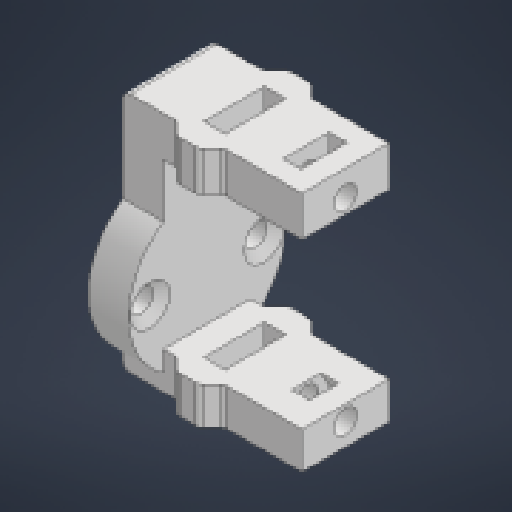
# Autodesk Inventor part: sg90 claw v2 holder
Saved by Autodesk Inventor 2026.1 (Build 301233020, 233B)
## iProperties
Created: 2025-05-12
Part Number: sg90 claw v2 holder
Material: 一般
Document SubType Name: Modeling
Designer: gavin
Density: 1 g/cm^3
Appearance: 預設
Author: gavin
## iProperties of the stored document sg90 claw v2 holder_3D 列印.ipt
Created: 2025-05-12
Part Number: sg90 claw v2 holder_3D 列印
Material: 一般
Document SubType Name: Modeling
Designer: gavin
Density: 1 g/cm^3
Appearance: 預設
Author: gavin
Autodesk Inventor part; units mm, degrees
ref_plane "YZ Plane" through (0, 0, 0) normal (1, 0, 0) x (0, 1, 0)
ref_plane "XZ Plane" through (0, 0, 0) normal (0, 1, 0) x (-1, 0, 0)
ref_plane "XY Plane" through (0, 0, 0) normal (0, 0, 1) x (1, 0, 0)
sketch "草圖1" plane through (0, 0, 0) normal (0, 0, 1) x (1, 0, 0)
  line L0 (-4.2926, 4.2164) -> (-4.2926, -0.635) projected
  line L1 (-4.2926, 4.2164) -> (-6.6548, 4.2164) projected
  line L2 (-6.6548, 4.2164) -> (-6.6548, -0.635) projected
  line L3 (-6.6548, -0.635) -> (-22.225, -0.635) projected
  line L4 (-22.225, -0.635) -> (-22.225, -3.6963) construction
  line L5 (-22.225, -3.6963) -> (-23.241, -3.6963) construction
  line L6 (-23.241, -3.6963) -> (-23.241, -19.2054) construction
  line L7 (-23.241, -19.2054) -> (-21.209, -19.2054) construction
  line L8 (-21.209, -19.2054) -> (-21.209, -21.9456) construction
  line L9 (-21.209, -21.9456) -> (-6.6548, -21.9456) projected
  line L10 (-6.6548, -26.797) -> (-6.6548, -21.9456) construction
  line L11 (-6.6548, -26.797) -> (-4.2926, -26.797) construction
  line L12 (-4.2926, -26.797) -> (-4.2926, -21.9456) projected
  line L13 (-4.2926, -21.9456) -> (0, -21.9456) projected
  line L14 (0, -16.4846) -> (0, -21.9456) projected
  line L15 (0, -0.635) -> (0, -16.4846) projected
  line L16 (0, -0.635) -> (-4.2926, -0.635) projected
  line L17 (-6.6548, -19.8311) -> (-6.6548, -2.7496) projected
  line L18 (-19.6088, -19.8311) -> (-6.6548, -19.8311) projected
  line L19 (-19.6088, -2.7496) -> (-19.6088, -19.8311) projected
  line L20 (-6.6548, -2.7496) -> (-19.6088, -2.7496) projected
  line L21 (-23.06, 0.2) -> (-12.0824, 0.2)
  line L22 (-6.8548, 4.8514) -> (-6.6548, 4.8514)
  line L23 (-4.0926, 4.4164) -> (-4.0926, -0.435)
  line L24 (-4.0926, -0.435) -> (0.2, -0.435)
  line L25 (0.2, -0.435) -> (0.2, -16.4846)
  line L26 (0.2, -16.4846) -> (0.2, -22.1456)
  line L27 (0.2, -22.1456) -> (-4.0926, -22.1456)
  line L28 (-4.0926, -22.1456) -> (-4.0926, -26.997)
  line L29 (-6.6548, -26.997) -> (-9.1539, -26.997)
  line L30 (-6.8548, -22.7806) -> (-22.044, -22.7806)
  line L31 (-22.044, -22.7806) -> (-22.044, -20.0404) construction
  line L32 (-22.044, -20.0404) -> (-24.076, -20.0404) construction
  line L33 (-24.076, -20.0404) -> (-24.076, -2.8613) construction
  line L34 (-24.076, -2.8613) -> (-23.06, -2.8613) construction
  line L35 (-23.06, -2.8613) -> (-23.06, 0.2) construction
  line L36 (-6.8548, 4.8514) -> (-31.7274, 4.8514)
  line L37 (-24.076, -11.4509) -> (-24.6908, -11.4509)
  line L38 (-31.7274, 4.8514) -> (-31.7274, -11.4509)
  line L39 (-23.06, 0.2) -> (-27.076, 0.2)
  line L40 (-27.076, 0.2) -> (-27.076, -11.4509)
  line L41 (-9.1539, -26.997) -> (-31.7274, -26.997)
  line L42 (-31.7274, -26.997) -> (-31.7274, -11.4509)
  line L43 (-27.076, -11.4509) -> (-27.076, -22.7806)
  line L44 (-27.076, -22.7806) -> (-22.044, -22.7806)
  line L45 (-6.6548, 4.8514) -> (-6.6548, 0.2)
  line L46 (-12.0824, 0.2) -> (-6.6548, 0.2)
  line L47 (-6.8548, -22.7806) -> (-6.6548, -22.7806)
  line L48 (-6.6548, -26.997) -> (-6.6548, -22.7806)
  line L49 (-6.6548, -22.5806) -> (-21.844, -22.5806)
  line L50 (-22.225, 0) -> (-6.6548, 0)
  line L51 (-6.6548, 4.8514) -> (-4.2926, 4.8514)
  point P0 (0, 0)
  point P1 (-5.4737, 4.8514)
  dimension "d4" = 3
  dimension "d6" = 4.6514
  dimension "d7" = 4.6514
  dimension "d37" = 0.2
  dimension "d38" = 0.2
  constraints: 62 end point, 7 horizontal, 5 perpendicular, 5 point on line, 3 vertical, 2 collinear, 2 midpoint, 1 horizontal alignment, 16 other
  measures "d4" distance between parallel lines of L40 L33
  measures "d6" distance between parallel lines of L39 L36
  measures "d7" distance between parallel lines of L38 L40
  measures "d37" distance between parallel lines of L50 L21
  measures "d38" distance between parallel lines of L49 L30
ref_plane "工作平面1" through (-23.241, -26.797, -12.192) normal (0, 0, -1) x (0, 1, 0)
extrude "擠出1" add sketch "草圖1" against normal up to surface (12.192 mm away) contours L2 L46 L21 L39 L40 L43 L44 L30 L47 L48 L29 L41 L42 L38 L36 L22 L45
sketch "草圖3" plane through (-31.7274, 4.8514, 0) normal (0, 1, 0) x (1, 0, 0)
  line L0 (25.0726, 12.192) -> (0, 12.192) projected
  line L1 (0, 0) -> (0, 12.192) projected
  line L2 (25.0726, 0) -> (0, 0) projected
  line L3 (25.0726, 0) -> (25.0726, 12.192) projected
  point P0 (31.7274, 0)
extrude "擠出3" add sketch "草圖3" along normal blind 1
sketch "草圖4" plane through (-31.7274, -26.997, 0) normal (0, -1, 0) x (1, 0, 0)
  line L0 (0, -12.192) -> (25.0726, -12.192) projected
  line L1 (0, 0) -> (25.0726, 0) projected
  line L2 (0, 0) -> (0, -12.192) projected
  line L3 (25.0726, 0) -> (25.0726, -12.192) projected
  point P0 (31.7274, 0)
extrude "擠出4" add sketch "草圖4" along normal blind 1
ref_plane "工作平面2" through (-9.6548, -22.7806, 0) normal (1, 0, 0) x (0, 0, -1)
sketch "草圖5" plane through (-9.6548, -22.7806, 0) normal (1, 0, 0) x (0, 0, -1)
  circle A0 centre (6.096, -2.086) radius 1.65 projected
  line L0 (4.4794, -4.886) -> (2.8628, -2.086)
  line L1 (2.8628, -2.086) -> (4.4794, 0.714)
  line L2 (4.4794, 0.714) -> (7.7126, 0.714)
  line L3 (7.7126, 0.714) -> (9.3292, -2.086)
  line L4 (9.3292, -2.086) -> (7.7126, -4.886)
  line L5 (7.7126, -4.886) -> (4.4794, -4.886)
  line L6 (2.8628, -2.086) -> (2.8628, -8.9822)
  line L7 (2.8628, -8.9822) -> (9.3292, -8.9822)
  line L8 (9.3292, -8.9822) -> (9.3292, -2.086)
  point P0 (0, 22.7806)
  dimension "d19" = 5.6
  constraints: 18 end point, 2 perpendicular, 1 coincident, 1 vertical, 13 other
  measures "d19" distance between parallel lines of L5 L2
extrude "擠出5" cut sketch "草圖5" against normal blind 2.5 contours A0 | L5 L4 L8 L7 L6 L0 | L0 L1 L2 L3 L4 L5
ref_plane "工作平面3" through (-31.7274, -11.0728, 0) normal (0, 1, 0) x (1, 0, 0)
mirror "鏡射1" about plane through (-31.7274, -11.0728, 0) normal (0, 1, 0) of "擠出5"
sketch "草圖10" plane through (-6.6548, -22.7806, 0) normal (1, 0, 0) x (0, 0, -1)
  circle A0 centre (6.096, 25.0666) radius 1.6 projected
  arc A1 (6.731, -3.8821) -> (5.461, -3.8821) centre (6.096, -2.086) ccw projected
  circle A2 centre (6.096, -2.086) radius 1.65
  circle A3 centre (6.096, 25.0666) radius 1.65
  point P0 (0, 22.7806)
  dimension "d39" = 3.3
  dimension "d40" = 3.3
  constraints: 2 centre point, 1 coincident
  measures "d39" diameter of A2
  measures "d40" diameter of A3
extrude "擠出10" cut sketch "草圖10" against normal blind 11 contours A0 | A2
fillet "圓角2" radius 1 1 edges at (-31.7274, 5.8514, -6.096)
sketch "草圖12" plane through (-31.7274, 5.8514, 0) normal (0, 1, 0) x (1, 0, 0)
  line L0 (1, 0) -> (1, 12.192) projected
  line L1 (1, 0) -> (25.0726, 0) projected
  line L2 (25.0726, 0) -> (25.0726, 12.192) projected
  line L3 (25.0726, 12.192) -> (1, 12.192) projected
  line L4 (19.5726, 9.3292) -> (22.0726, 9.3292) projected
  line L5 (22.0726, 9.3292) -> (22.0726, 2.8628) projected
  line L6 (22.0726, 2.8628) -> (19.5726, 2.8628) projected
  line L7 (19.5726, 2.8628) -> (19.5726, 9.3292) projected
  line L8 (12.4726, 10.346) -> (9.4726, 10.346)
  line L9 (9.4726, 10.346) -> (9.4726, 1.846)
  line L10 (9.4726, 1.846) -> (12.4726, 1.846)
  line L11 (12.4726, 1.846) -> (12.4726, 10.346)
  point P0 (31.7274, 0)
  dimension "d47" = 3
  dimension "d48" = 8.5
  dimension "d49" = 12.192
  dimension "d50" = 1.846
  dimension "d51" = 12.6
  constraints: 8 end point, 2 parallel, 1 horizontal, 1 perpendicular
  measures "d47" distance of L9.end L10.end
  measures "d48" distance of L8.end L9.end
  measures "d49" distance of L1.end L2.end
  measures "d50" distance between parallel lines of L8 L3
  measures "d51" distance between parallel lines of L2 L11
extrude "擠出12" cut sketch "草圖12" against normal up to surface (5.6514 mm away) contours L11 L10 L9 L8
sketch "草圖13" plane through (-31.7274, 5.8514, 0) normal (0, 1, 0) x (1, 0, 0)
  line L0 (9.4726, 10.346) -> (12.4726, 10.346) projected
  line L1 (12.4726, 10.346) -> (12.4726, 1.846) projected
  line L2 (12.4726, 1.846) -> (9.4726, 1.846) projected
  line L3 (9.4726, 1.846) -> (9.4726, 10.346) projected
  line L4 (1, 0) -> (1, 12.192) projected
  line L5 (1, 0) -> (25.0726, 0) projected
  line L6 (25.0726, 0) -> (25.0726, 12.192) projected
  line L7 (25.0726, 12.192) -> (1, 12.192) projected
  line L8 (19.5726, 9.3292) -> (22.0726, 9.3292) projected
  line L9 (22.0726, 9.3292) -> (22.0726, 2.8628) projected
  line L10 (22.0726, 2.8628) -> (19.5726, 2.8628) projected
  line L11 (19.5726, 2.8628) -> (19.5726, 9.3292) projected
  line L12 (12.3526, 13.992) -> (9.3526, 13.992)
  line L13 (9.3526, 13.992) -> (7.5526, 12.192)
  line L14 (12.3526, 13.992) -> (14.1526, 12.192)
  line L15 (25.0726, 6.096) -> (20.8226, 6.096) construction
  line L16 (12.3526, -1.8) -> (9.3526, -1.8)
  line L17 (9.3526, -1.8) -> (7.5526, 0)
  line L18 (12.3526, -1.8) -> (14.1526, 0)
  point P0 (31.7274, 0)
  dimension "d54" = 135
  dimension "d55" = 135
  dimension "d56" = 1.8
  constraints: 14 end point, 4 symmetric about line, 2 horizontal, 2 point on line, 1 midpoint
  measures "d54" angle of L12 L14
  measures "d55" angle of L13 L12
  measures "d56" distance between parallel lines of L7 L12
extrude "擠出13" add sketch "草圖13" against normal up to surface (5.6514 mm away) contours L5 L18 L16 L17 | L13 L12 L14 L7
fillet "圓角3" radius 1 8 edges at (-17.5748, 3.0257, 0) (-19.3748, 3.0257, 1.8) (-22.3748, 3.0257, 1.8) (-24.1748, 3.0257, 0) (-17.5748, 3.0257, -12.192) (-19.3748, 3.0257, -13.992) (-22.3748, 3.0257, -13.992) (-24.1748, 3.0257, -12.192)
sketch "草圖14" plane through (-31.7274, -27.997, 0) normal (0, -1, 0) x (1, 0, 0)
  line L0 (12.4726, -10.346) -> (9.4726, -10.346) projected
  line L1 (9.4726, -10.346) -> (9.4726, -1.846) projected
  line L2 (9.4726, -1.846) -> (12.4726, -1.846) projected
  line L3 (12.4726, -1.846) -> (12.4726, -10.346) projected
  line L4 (22.0726, -7.8737) -> (19.5726, -7.8737) projected
  line L5 (19.5726, -7.8737) -> (19.5726, -4.3183) projected
  line L6 (19.5726, -4.3183) -> (22.0726, -4.3183) projected
  line L7 (22.0726, -4.3183) -> (22.0726, -7.8737) projected
  arc A0 (9.0597, -13.6991) -> (9.7668, -13.992) centre (9.7668, -12.992) ccw projected
  line L8 (11.9384, -13.992) -> (9.7668, -13.992) projected
  arc A1 (11.9384, -13.992) -> (12.6455, -13.6991) centre (11.9384, -12.992) ccw projected
  line L9 (13.8597, -12.4849) -> (12.6455, -13.6991) projected
  arc A2 (14.5668, -12.192) -> (13.8597, -12.4849) centre (14.5668, -13.192) ccw projected
  line L10 (14.5668, -12.192) -> (25.0726, -12.192) projected
  line L11 (25.0726, 0) -> (25.0726, -12.192) projected
  line L12 (14.5668, 0) -> (25.0726, 0) projected
  arc A3 (13.8597, 0.2929) -> (14.5668, 0) centre (14.5668, 1) ccw projected
  line L13 (12.6455, 1.5071) -> (13.8597, 0.2929) projected
  arc A4 (12.6455, 1.5071) -> (11.9384, 1.8) centre (11.9384, 0.8) ccw projected
  line L14 (9.7668, 1.8) -> (11.9384, 1.8) projected
  arc A5 (9.7668, 1.8) -> (9.0597, 1.5071) centre (9.7668, 0.8) ccw projected
  line L15 (7.8455, 0.2929) -> (9.0597, 1.5071) projected
  arc A6 (7.1384, 0) -> (7.8455, 0.2929) centre (7.1384, 1) ccw projected
  line L16 (4.6514, 0) -> (7.1384, 0) projected
  line L17 (4.6514, 0) -> (4.6514, -12.192) projected
  line L18 (4.6514, -12.192) -> (7.1384, -12.192) projected
  arc A7 (7.8455, -12.4849) -> (7.1384, -12.192) centre (7.1384, -13.192) ccw projected
  line L19 (9.0597, -13.6991) -> (7.8455, -12.4849) projected
  point P0 (31.7274, 0)
extrude "擠出14" cut sketch "草圖14" against normal up to surface (5.2164 mm away) contours L0 L1 L2 L3
sketch "草圖15" plane through (-31.7274, -27.997, 0) normal (0, -1, 0) x (1, 0, 0)
  line L0 (12.4726, -10.346) -> (9.4726, -10.346) projected
  line L1 (9.4726, -10.346) -> (9.4726, -1.846) projected
  line L2 (9.4726, -1.846) -> (12.4726, -1.846) projected
  line L3 (12.4726, -1.846) -> (12.4726, -10.346) projected
  line L4 (22.0726, -7.8737) -> (19.5726, -7.8737) projected
  line L5 (19.5726, -7.8737) -> (19.5726, -4.3183) projected
  line L6 (19.5726, -4.3183) -> (22.0726, -4.3183) projected
  line L7 (22.0726, -4.3183) -> (22.0726, -7.8737) projected
  arc A0 (9.0597, -13.6991) -> (9.7668, -13.992) centre (9.7668, -12.992) ccw projected
  line L8 (11.9384, -13.992) -> (9.7668, -13.992) projected
  arc A1 (11.9384, -13.992) -> (12.6455, -13.6991) centre (11.9384, -12.992) ccw projected
  line L9 (13.8597, -12.4849) -> (12.6455, -13.6991) projected
  arc A2 (14.5668, -12.192) -> (13.8597, -12.4849) centre (14.5668, -13.192) ccw projected
  line L10 (14.5668, -12.192) -> (25.0726, -12.192) projected
  line L11 (25.0726, 0) -> (25.0726, -12.192) projected
  line L12 (14.5668, 0) -> (25.0726, 0) projected
  arc A3 (13.8597, 0.2929) -> (14.5668, 0) centre (14.5668, 1) ccw projected
  line L13 (12.6455, 1.5071) -> (13.8597, 0.2929) projected
  arc A4 (12.6455, 1.5071) -> (11.9384, 1.8) centre (11.9384, 0.8) ccw projected
  line L14 (9.7668, 1.8) -> (11.9384, 1.8) projected
  arc A5 (9.7668, 1.8) -> (9.0597, 1.5071) centre (9.7668, 0.8) ccw projected
  line L15 (7.8455, 0.2929) -> (9.0597, 1.5071) projected
  arc A6 (7.1384, 0) -> (7.8455, 0.2929) centre (7.1384, 1) ccw projected
  line L16 (4.6514, 0) -> (7.1384, 0) projected
  line L17 (4.6514, 0) -> (4.6514, -12.192) projected
  line L18 (4.6514, -12.192) -> (7.1384, -12.192) projected
  arc A7 (7.8455, -12.4849) -> (7.1384, -12.192) centre (7.1384, -13.192) ccw projected
  line L19 (9.0597, -13.6991) -> (7.8455, -12.4849) projected
  line L20 (14.5668, 0) -> (7.1384, 0)
  line L21 (25.0726, 0) -> (4.6514, 0) projected
  line L22 (14.5668, -12.192) -> (7.1384, -12.192)
  line L23 (25.0726, -12.192) -> (4.6514, -12.192) projected
  point P0 (31.7274, 0)
  constraints: 4 end point, 2 point on circle
extrude "擠出15" add sketch "草圖15" against normal up to surface (5.2164 mm away) contours L19 A7 L22 A2 L9 A1 L8 A0 | A6 L15 A5 L14 A4 L13 A3 L20
sketch "草圖16" plane through (-27.076, -22.7806, 0) normal (1, 0, 0) x (0, 0, -1)
  line L0 (12.192, 0) -> (12.192, 22.9806) projected
  line L1 (0, 22.9806) -> (12.192, 22.9806) projected
  line L2 (0, 0) -> (0, 22.9806) projected
  line L3 (0, 0) -> (12.192, 0) projected
  point P0 (0, 22.7806)
extrude "擠出16" add sketch "草圖16" along normal blind 1
sketch "草圖17" plane through (-31.7274, -27.997, -12.192) normal (-1, 0, 0) x (0, 0, 1)
  circle A0 centre (6.096, 11.5124) radius 1.225 projected
  circle A1 centre (6.096, 11.5124) radius 11
  point P0 (12.192, 27.997)
  dimension "d66" = 22
  constraints: 1 centre point, 1 coincident
  measures "d66" diameter of A1
extrude "擠出17" add sketch "草圖17" against normal up to surface (5.6514 mm away) contours A0 | A1
sketch "草圖18" plane through (-31.7274, -27.997, -12.192) normal (-1, 0, 0) x (0, 0, 1)
  arc A0 (12.192, 2.356) -> (12.192, 20.6688) centre (6.096, 11.5124) ccw projected
  circle A1 centre (6.096, 11.5124) radius 8 construction
  circle A2 centre (14.096, 11.5124) radius 1.6
  circle A3 centre (-1.904, 11.5124) radius 1.6
  point P0 (12.192, 27.997)
  dimension "d69" = 16
  dimension "d70" = 3.2
  dimension "d71" = 3.2
  constraints: 3 centre point, 2 point on circle, 1 coincident
  measures "d69" diameter of A1
  measures "d70" diameter of A2
  measures "d71" diameter of A3
extrude "擠出18" cut sketch "草圖18" against normal blind 10
fillet "圓角4" radius 1 1 edges at (-31.7274, -27.997, -6.096)
chamfer "Chamfer1" distance 1.2 angle 45 2 edges at (-26.076, -16.4846, 0.304) (-26.076, -16.4846, -15.696)
equation "\"d7\" = d6"
equation "\"d50\" = -0.5 * d48 + 0.5 * d49"
